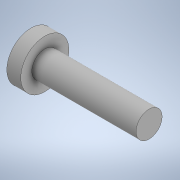
# Autodesk Inventor part: M3x12
Saved by Autodesk Inventor 2021 (Build 250183000, 183)
## iProperties
Created: 2024-03-24
Part Number: M3x12
Material: Generic
Document SubType Name: Modeling
Designer: Lukas
Density: 1 g/cm^3
Appearance: Default
Author: Lukas
Autodesk Inventor part; units mm, degrees
ref_plane "YZ Plane" through (0, 0, 0) normal (1, 0, 0) x (0, 1, 0)
ref_plane "XZ Plane" through (0, 0, 0) normal (0, 1, 0) x (-1, 0, 0)
ref_plane "XY Plane" through (0, 0, 0) normal (0, 0, 1) x (1, 0, 0)
sketch "Sketch1" plane through (0, 0, 0) normal (0, 0, 1) x (1, 0, 0)
  line L0 (0, 0) -> (-6.8, 0)
  line L1 (-6.8, 0) -> (-6.8, 2.775)
  line L2 (-6.8, 2.775) -> (-5.2, 2.775)
  line L3 (-5.2, 2.775) -> (-5.2, 1.5)
  line L4 (-5.2, 1.5) -> (6.8, 1.5)
  line L5 (6.8, 1.5) -> (6.8, 0)
  line L6 (6.8, 0) -> (0, 0)
  dimension "d0" = 12
  dimension "d1" = 2.775
  dimension "d2" = 1.6
  dimension "d3" = 1.5
  constraints: 14 end point, 6 perpendicular, 1 collinear, 1 horizontal, 1 point on line
  measures "d0" distance between parallel lines of L5 L3
  measures "d1" distance of L0.end L1.end
  measures "d2" distance of L1.end L2.end
  measures "d3" distance of L4.end L5.end
revolve "Revolution1" add sketch "Sketch1" angle 360 about axis through (0, 0, 0) along (-1, 0, 0)
sketch "Sketch2" plane through (-6.8, 0, 0) normal (-1, 0, 0) x (0, 0, 1)
  line L0 (-1.1547, 0) -> (-0.5774, 1)
  line L1 (-0.5774, 1) -> (0.5774, 1)
  line L2 (0.5774, 1) -> (1.1547, 0)
  line L3 (1.1547, 0) -> (0.5774, -1)
  line L4 (0.5774, -1) -> (-0.5774, -1)
  line L5 (-0.5774, -1) -> (-1.1547, 0)
  point P0 (0, 0)
  point P1 (0, 0)
  dimension "d5" = 2
  constraints: 12 end point, 1 coincident, 1 horizontal alignment, 13 other
  measures "d5" distance between parallel lines of L4 L1
extrude "Extrusion1" cut sketch "Sketch2" against normal blind 1.5
body "Solid1"
